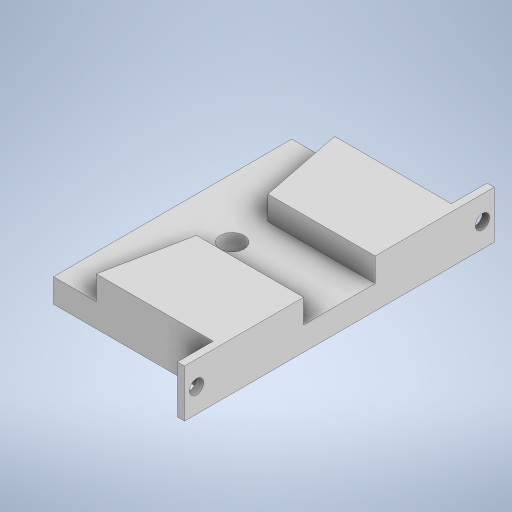
# Autodesk Inventor part: Стенка
Saved by Autodesk Inventor 2023 (Build 270158000, 158)
## iProperties
Created: 2022-04-28
Part Number: Стенка
Material: Типовые
Document SubType Name: Modeling
Designer: User
Density: 1 g/cm^3
Appearance: По умолчанию
Author: User
Autodesk Inventor part; units mm, degrees
ref_plane "YZ Plane" through (0, 0, 0) normal (1, 0, 0) x (0, 1, 0)
ref_plane "XZ Plane" through (0, 0, 0) normal (0, 1, 0) x (-1, 0, 0)
ref_plane "XY Plane" through (0, 0, 0) normal (0, 0, 1) x (1, 0, 0)
sketch "Эскиз1" plane through (0, 0, 0) normal (0, 1, 0) x (-1, 0, 0)
  line L0 (0, 0) -> (70, 0)
  line L1 (70, 0) -> (70, -100)
  line L2 (70, -100) -> (0, -100)
  line L3 (0, -100) -> (0, 0)
  dimension "d0" = 70
  dimension "d1" = 100
  constraints: 8 end point, 2 parallel, 1 horizontal, 1 perpendicular
  measures "d0" distance of L1.end L2.end
  measures "d1" distance of L0.end L1.end
extrude "Выдавливание1" add sketch "Эскиз1" along normal blind 10
sketch "Эскиз2" plane through (0, 10, 0) normal (0, 1, 0) x (1, 0, 0)
  line L0 (0, 0) -> (0, 100) projected
  line L1 (0, 50) -> (-45, 50)
  circle A0 centre (-45, 50) radius 5
  line L2 (0, 50) -> (0, 65)
  line L3 (0, 65) -> (-45, 65)
  line L4 (0, 50) -> (0, 35)
  line L5 (0, 35) -> (-45, 35)
  line L6 (-45, 50) -> (-70, 50)
  line L7 (-70, 100) -> (-70, 0) projected
  line L8 (-45, 50) -> (5, 50) construction
  line L9 (-45, 50) -> (-50.0759, 24.6207)
  line L10 (-45, 50) -> (15, 50) construction
  line L11 (-50.0759, 24.6207) -> (-50.0759, 75.3793)
  line L12 (-45, 50) -> (-50.0759, 75.3793)
  circle A1 centre (-45, 50) radius 9
  line L13 (-45, 65) -> (-52, 100)
  line L14 (-45, 35) -> (-52, 0)
  line L15 (-52, 0) -> (0, 0)
  line L16 (0, 0) -> (0, 100)
  line L17 (0, 100) -> (-52, 100)
  dimension "d4" = 45
  dimension "d5" = 10
  dimension "d6" = 15
  dimension "d7" = 15
  dimension "d12" = 157.38
  dimension "d13" = 18
  dimension "d18" = 52
  dimension "d19" = 45
  constraints: 32 end point, 4 perpendicular, 3 horizontal, 2 centre point, 2 coincident, 2 equal length, 2 midpoint, 2 parallel, 2 point on line, 1 vertical
  measures "d4" distance of L1.start L1.end
  measures "d5" diameter of A0
  measures "d6" distance of L1.start L2.end
  measures "d7" distance of L1.start L4.end
  measures "d12" angle of L9 L12
  measures "d13" diameter of A1
  measures "d18" distance of L0.end L13.end
  measures "d19" distance of L2.end L3.end
extrude "Выдавливание2" add sketch "Эскиз2" along normal blind 10 contours L15 L14 L5 L0 | L3 L13 L17 L0
extrude "Выдавливание3" cut sketch "Эскиз2" against normal blind 42.5 contours A0 L9 L1 | L1 L12 A0 | L9 A0 L6 | L6 A0 L12
sketch "Эскиз3" plane through (0, 0, 0) normal (0, -1, 0) x (1, 0, 0)
  circle A0 centre (-45, -50) radius 5 projected
  line L0 (-45, -50) -> (-15, -50)
  circle A1 centre (-15, -50) radius 6
  point P0 (0, 0)
  dimension "d20" = 30
  dimension "d21" = 12
  constraints: 2 end point, 1 centre point, 1 coincident, 1 horizontal
  measures "d20" distance of L0.start L0.end
  measures "d21" diameter of A1
extrude "Выдавливание4" cut sketch "Эскиз3" against normal blind 3 contours A1
chamfer "Фаска1" distance 1 angle 45 1 edges at (-21, 0, -50)
sketch "Эскиз4" plane through (0, 0, 0) normal (1, 0, 0) x (0, 0, -1)
  line L0 (0, 0) -> (0, 20) projected
  line L1 (0, 0) -> (-15, 0)
  line L2 (-15, 0) -> (-15, 20)
  line L3 (-15, 20) -> (0, 20)
  line L4 (0, 20) -> (0, 0)
  line L5 (100, 0) -> (100, 20) projected
  line L6 (100, 0) -> (115, 0)
  line L7 (115, 0) -> (115, 20)
  line L8 (115, 20) -> (100, 20)
  line L9 (100, 20) -> (100, 0)
  line L10 (115, 20) -> (110, 20)
  line L11 (110, 20) -> (110, 10)
  line L12 (110, 10) -> (115, 10)
  line L13 (115, 10) -> (115, 20)
  line L14 (-15, 20) -> (-10, 20)
  line L15 (-10, 20) -> (-10, 10)
  line L16 (-10, 10) -> (-15, 10)
  line L17 (-15, 10) -> (-15, 20)
  circle A0 centre (-10, 10) radius 3
  circle A1 centre (110, 10) radius 3
  line L18 (100, 20) -> (0, 20)
  dimension "d27" = 15
  dimension "d28" = 15
  dimension "d29" = 5
  dimension "d30" = 10
  dimension "d31" = 5
  dimension "d32" = 10
  dimension "d33" = 6
  dimension "d34" = 6
  constraints: 34 end point, 8 parallel, 5 perpendicular, 4 horizontal, 2 centre point, 2 coincident, 1 point on line
  measures "d27" distance of L2.end L3.end
  measures "d28" distance of L8.end L7.end
  measures "d29" distance of L12.end L11.end
  measures "d30" distance of L11.end L10.end
  measures "d31" distance of L15.end L16.end
  measures "d32" distance of L14.end L15.end
  measures "d33" diameter of A0
  measures "d34" diameter of A1
extrude "Выдавливание5" add sketch "Эскиз4" against normal blind 3 contours L1 L2 L16 A0 L15 L3 L0 | L15 A0 L16 L2 L3 | L5 L8 L11 A1 L12 L7 L6 | L8 L7 L12 A1 L11
